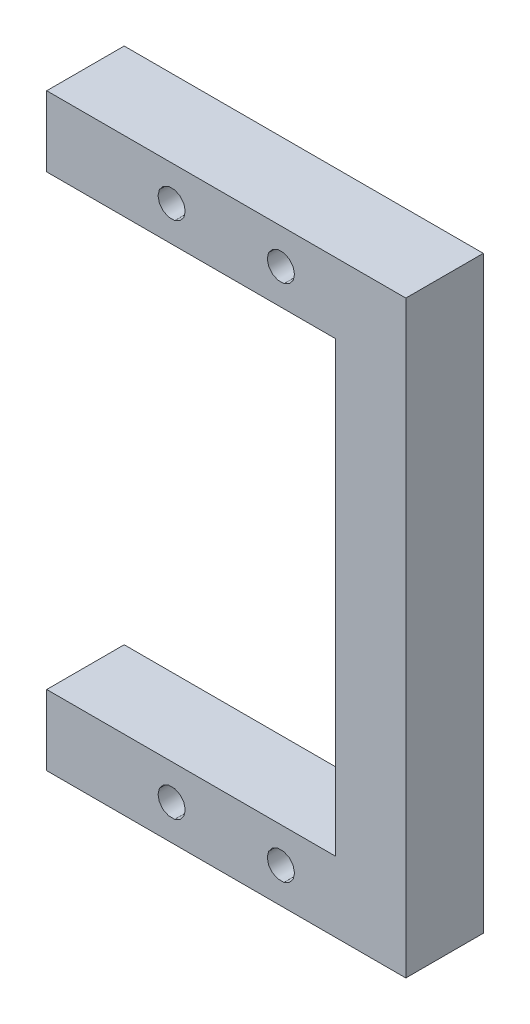
# Autodesk Inventor part: New Flipper
Saved by Autodesk Inventor 2015 (Build 190159000, 159)
## iProperties
Created: 2015-02-27
Part Number: New Flipper
Material: Generic
Document SubType Name: Modeling
Designer: jesse
Density: 1 g/cm^3
Appearance: Default
Author: jesse
Autodesk Inventor part; units mm, degrees
ref_plane "YZ Plane" through (0, 0, 0) normal (1, 0, 0) x (0, 1, 0)
ref_plane "XZ Plane" through (0, 0, 0) normal (0, 1, 0) x (-1, 0, 0)
ref_plane "XY Plane" through (0, 0, 0) normal (0, 0, 1) x (1, 0, 0)
sketch "Sketch1" plane through (0, 0, 0) normal (0, 0, 1) x (1, 0, 0)
  line L0 (0, 0) -> (0, 58.7756)
  line L1 (0, 58.7756) -> (28.6512, 58.7756)
  line L2 (28.6512, 58.7756) -> (28.6512, 0)
  line L3 (28.6512, 0) -> (0, 0)
  line L4 (-9.2202, 67.9958) -> (-9.2202, -9.2202)
  line L5 (-9.2202, -9.2202) -> (37.8714, -9.2202)
  line L6 (37.8714, -9.2202) -> (37.8714, 67.9958)
  line L7 (37.8714, 67.9958) -> (-9.2202, 67.9958)
  dimension "d0" = 28.6512
  dimension "d1" = 58.7756
  dimension "d2" = 9.2202
  constraints: 16 end point, 4 perpendicular, 2 vertical, 3 other
  measures "d0" distance of L0.end L1.end
  measures "d1" distance of L1.end L2.end
  measures "d2" distance between parallel lines of L0 L4
extrude "Extrusion1" add sketch "Sketch1" along normal blind 10.16
sketch "Sketch2" plane through (0, 0, 10.16) normal (0, 0, 1) x (1, 0, 0)
  line L0 (0, 58.7756) -> (28.6512, 58.7756) projected
  line L1 (28.6512, 58.7756) -> (28.6512, 0) projected
  line L2 (28.6512, 0) -> (0, 0) projected
  line L3 (0, 0) -> (0, 58.7756) projected
  line L4 (-9.2202, 67.9958) -> (-9.2202, -9.2202) projected
  line L5 (-9.2202, -9.2202) -> (37.8714, -9.2202) projected
  line L6 (37.8714, -9.2202) -> (37.8714, 67.9958) projected
  line L7 (37.8714, 67.9958) -> (-9.2202, 67.9958) projected
  line L8 (14.3256, 67.9958) -> (14.3256, 58.7756) construction
  line L9 (0, 58.7756) -> (28.6512, 58.7756) construction
  line L10 (14.3256, 63.3857) -> (28.6512, 63.3857) construction
  line L11 (14.3256, 63.3857) -> (0, 63.3857) construction
  circle A0 centre (7.1628, 63.3857) radius 1.7859
  circle A1 centre (21.4884, 63.3857) radius 1.7859
  line L12 (14.3256, 0) -> (14.3256, -9.2202) construction
  line L13 (-9.2202, -9.2202) -> (37.8714, -9.2202) construction
  line L14 (14.3256, -4.6101) -> (0, -4.6101) construction
  line L15 (14.3256, -4.6101) -> (28.6512, -4.6101) construction
  circle A2 centre (7.1628, -4.6101) radius 1.7859
  circle A3 centre (21.4884, -4.6101) radius 1.7859
  dimension "d5" = 3.5719
  dimension "d6" = 3.5719
  dimension "d7" = 3.5719
  dimension "d8" = 3.5719
  constraints: 12 end point, 10 midpoint, 4 centre point, 3 horizontal, 1 point on line
  measures "d5" diameter of A0
  measures "d6" diameter of A1
  measures "d7" diameter of A2
  measures "d8" diameter of A3
extrude "Extrusion2" cut sketch "Sketch2" against normal through all contours A0 | A1 | A2 | A3
sketch "Sketch3" plane through (0, 0, 10.16) normal (0, 0, 1) x (1, 0, 0)
  circle A0 centre (7.1628, -4.6101) radius 1.7859 projected
  circle A1 centre (7.1628, 63.3857) radius 1.7859 projected
  circle A2 centre (21.4884, 63.3857) radius 1.7859 projected
  circle A3 centre (21.4884, -4.6101) radius 1.7859 projected
  line L0 (0, 58.7756) -> (28.6512, 58.7756) projected
  line L1 (28.6512, 58.7756) -> (28.6512, 0) projected
  line L2 (28.6512, 0) -> (0, 0) projected
  line L3 (0, 0) -> (0, 58.7756) projected
  line L4 (-9.2202, 67.9958) -> (-9.2202, -9.2202) projected
  line L5 (-9.2202, -9.2202) -> (37.8714, -9.2202) projected
  line L6 (37.8714, -9.2202) -> (37.8714, 67.9958) projected
  line L7 (37.8714, 67.9958) -> (-9.2202, 67.9958) projected
  line L8 (-9.2202, 67.9958) -> (-9.2202, -9.2202) projected
  line L9 (0, 58.7756) -> (-9.2202, 58.7756)
  line L10 (-9.2202, 58.7756) -> (-9.2202, 0)
  line L11 (-9.2202, 0) -> (0, 0)
  line L12 (0, 0) -> (0, 58.7756)
  constraints: 8 end point, 2 parallel, 1 horizontal, 1 perpendicular, 1 point on line
extrude "Extrusion3" cut sketch "Sketch3" against normal through all contours L3 L11 L4 L9
body "Solid1"
